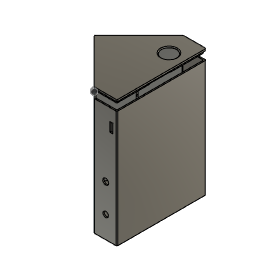
campanion enclosure (Autodesk Fusion 360 design; units mm, degrees)
Autodesk Fusion 360 part; units mm, degrees
note: some values were not read from the file. Chosen so that the rebuilt part matches the saved one: which face or edge a step refers to. Set by a fixed rule: which sketch regions a step uses.
sketch "Sketch1" plane through (0, 0, 0) normal (1, 0, 0) x (0, 1, 0)
  line L0 (0, 0) -> (51.6188, -51.6188)
  line L1 (0, 0) -> (73, 0) construction
  line L2 (0, 0) -> (0, -106.5194)
  line L3 (51.6188, -51.6188) -> (51.6188, -76.6188)
  line L4 (51.6188, -76.6188) -> (0, -76.6188)
  line L5 (0, 0) -> (-51.6188, -51.6188)
  line L6 (-51.6188, -51.6188) -> (-51.6188, -76.6188)
  line L7 (-51.6188, -76.6188) -> (0, -76.6188)
  line L8 (0, 2.1213) -> (53.1188, -50.9975)
  line L9 (53.1188, -50.9975) -> (53.1188, -78.1188)
  line L10 (53.1188, -78.1188) -> (0, -78.1188)
  line L11 (0, 2.1213) -> (-53.1188, -50.9975)
  line L12 (-53.1188, -50.9975) -> (-53.1188, -78.1188)
  line L13 (-53.1188, -78.1188) -> (0, -78.1188)
  dimension "d6" = 45
  dimension "d7" = 73
  dimension "d8" = 25
  constraint horizontal L1
  constraint coincident L0.start L1.start
  constraint perpendicular L1 L2
  constraint vertical L3
  constraint coincident L2 L4.end
  constraint perpendicular L2 L4
  constraint symmetric L0.start L2 L1.start
  constraint symmetric L0.end L2 L5.end
  constraint symmetric L2 L3.end L6.end
  constraint symmetric L2 L4.end L7.end
  constraint parallel L0 L8
  constraint parallel L3 L9
  constraint parallel L4 L10
  constraint parallel L5 L11
  constraint parallel L6 L12
  constraint parallel L7 L13
  measures "d6" angle of L0 L1
  measures "d7" distance of L0.start L0.end
  measures "d8" distance of L0.end L3.end
extrude "Extrude1" add sketch "Sketch1" along normal blind 124 makes body 1
sketch "Sketch3" plane through (0, -53.6188, 0) normal (0, -1, 0) x (1, 0, 0)
  line L0 (0, -78.6188) -> (124, -78.6188)
  line L1 (124, -78.6188) -> (124, -50.7904)
  line L2 (124, -50.7904) -> (0, -50.7904)
  line L3 (122.913, -78.6188) -> (122.913, -64.7048)
  line L4 (122.913, -64.7048) -> (124, -64.7046)
  line L5 (122.913, -64.7048) -> (-1, -64.7047)
  circle A0 centre (21.121, -64.7047) radius 3.25
  circle A1 centre (54.96, -64.7181) radius 3.5
  line L6 (124, -64.7046) -> (104.5, -64.7046)
  line L7 (-1, -64.7047) -> (18.5, -64.7047)
  line L8 (0, -50.7904) -> (0, -78.6188)
  dimension "d17" = 27.8284
  dimension "d18" = 13.914
  dimension "d19" = 6.5
  dimension "d20" = 7
  dimension "d21" = 19.5
  dimension "d22" = 19.5
  constraint coincident L0 L3.start
  constraint perpendicular L0 L3
  constraint midpoint L1 L4.end
  constraint coincident L5 A0.centre
  constraint coincident L4 A1.centre
  constraint perpendicular L1 L6
  measures "d17" distance of L0 L2
  measures "d18" distance of L3.start L3.end
  measures "d19" diameter of A0
  measures "d20" diameter of A1
  measures "d21" distance of L4.end L6.end
  measures "d22" distance of L5.end L7.end
extrude "Extrude3" cut sketch "Sketch3" against normal blind 2 contours L5 A0 L7 | L5 A0 L7 | L5 A1 | L5 A1 bodies 1
sketch "Sketch4" plane through (0, -1.4142, 1.4142) normal (0, -0.707107, 0.707107) x (1, 0, 0)
  line L0 (0, -73.8284) -> (124, -73.8284)
  line L1 (124, -73.8284) -> (124, 2)
  line L2 (124, 2) -> (0, 2)
  line L3 (1.4348, -7.7738) -> (77.4348, -7.7738)
  line L4 (77.4348, -7.7738) -> (77.4348, -62.7738)
  line L5 (77.4348, -62.7738) -> (1.4348, -62.7738)
  line L6 (1.4348, -62.7738) -> (1.4348, -7.7738)
  line L7 (0, 2) -> (0, -73.8284)
  dimension "d25" = 76
  dimension "d26" = 55
  constraint horizontal L3
  constraint vertical L4
  constraint horizontal L5
  constraint vertical L6
  measures "d25" distance of L3.start L3.end
  measures "d26" distance of L3.start L5.end
extrude "Extrude4" cut sketch "Sketch4" against normal blind 2 contours L3 L4 L5 L6 bodies 1
extrude "Extrude5" add 1 faces at (0, -17.2063, -77.6188) along direction (-1, 0, 0) blind 3 on bodies 1 bodies 1
ref_plane "WorkPlane1" through (-3, 0, 0) normal (1, 0, 0) x (0, 1, 0)
sketch "Sketch6" plane through (-3, 0, 0) normal (1, 0, 0) x (0, 1, 0)
  line L0 (0, 1.066) -> (-52.4214, -50.8821)
  line L1 (-52.4214, -50.8821) -> (-52.4214, -77.9172)
  line L2 (-52.4214, -77.9172) -> (52.8588, -77.9172)
  line L3 (52.8588, -77.9172) -> (52.8588, -50.8821)
  line L4 (52.8588, -50.8821) -> (0, 1.066)
  constraint vertical L1
  constraint perpendicular L1 L2
  constraint perpendicular L2 L3
extrude "Extrude7" add 1 faces at (-3, -17.2063, -77.6188) along direction (-1, 0, 0) blind 2 on bodies 1 bodies 1
extrude "Extrude8" add sketch "Sketch6" against normal blind 2 bodies 1
ref_plane "WorkPlane2" through (59.5, -1.4571, -49.5404) normal (0, -0.707107, 0.707107) x (0, -0.707107, -0.707107)
sketch "Sketch7" plane through (49.5, -1.3536, -49.4368) normal (0, -0.707107, 0.707107) x (0, -0.707107, -0.707107)
  line L0 (-37.4062, -54.4523) -> (37.8896, -54.4523)
  line L1 (37.8896, -54.4523) -> (37.8896, 74.4408)
  line L2 (37.8896, 74.4408) -> (-37.4062, 74.4408)
  line L3 (-37.4062, 74.4408) -> (-37.4062, -54.4523)
  constraint horizontal L0
  constraint vertical L1
  constraint horizontal L2
  constraint vertical L3
extrude "Extrude12" add 1 faces at (124, -17.2063, -77.6188) along direction (1, 0, 0) blind 10 on bodies 1 bodies 1
ref_plane "WorkPlane3" through (134, 0, 0) normal (1, 0, 0) x (0, 1, 0)
sketch "Sketch8" plane through (134, 0, 0) normal (1, 0, 0) x (0, 1, 0)
  line L0 (-27.0492, -74.4051) -> (-30.0877, -77.4712)
  line L1 (-30.0877, -77.4712) -> (-28.0645, -78.0602)
  line L2 (-25.4859, -75.6609) -> (-27.3218, -77.4968)
  line L3 (-27.3218, -77.4968) -> (-28.0645, -78.0602)
  line L4 (-27.0492, -74.4051) -> (-25.4859, -75.6609)
sketch "Sketch9" plane through (49.5, -1.3536, -49.4368) normal (0, -0.707107, 0.707107) x (0, -0.707107, -0.707107)
sketch "Sketch10" plane through (49.5, -1.3536, -49.4368) normal (0, -0.707107, 0.707107) x (0, -0.707107, -0.707107)
  line L0 (37.1723, -20.8219) -> (40.3659, -20.8219)
  line L1 (40.3659, -20.8219) -> (40.3659, -0.7333)
  line L2 (40.3659, -0.7333) -> (37.1723, -0.7333)
  line L3 (37.1723, -0.7333) -> (37.1723, -20.8219)
  line L4 (37.1723, 35.5294) -> (40.3659, 35.5294)
  line L5 (40.3659, 35.5294) -> (40.3659, 52.3215)
  line L6 (40.3659, 52.3215) -> (37.1723, 52.3215)
  line L7 (37.1723, 52.3215) -> (37.1723, 35.5294)
  constraint horizontal L0
  constraint vertical L1
  constraint horizontal L2
  constraint vertical L3
  constraint horizontal L4
  constraint vertical L5
  constraint horizontal L6
  constraint vertical L7
extrude "Extrude11" add sketch "Sketch10" along normal blind 18 bodies 1
fillet "Fillet1" radius 1 16 edges at (38.7224, -40.3663, -62.9937) (48.7667, -34.0023, -69.3576) (48.7667, -36.941, -70.9353) (48.7667, -41.4954, -64.1228) (38.7224, -42.6245, -65.2519) (28.6781, -41.4954, -64.1228) (28.6781, -36.941, -70.9353) (28.6781, -34.0023, -69.3576) (85.0294, -34.0023, -69.3576) (85.0294, -36.941, -70.9353) (85.0294, -41.4954, -64.1228) (93.4254, -42.6245, -65.2519) (93.4254, -40.3663, -62.9937) (101.8215, -34.0023, -69.3576) (101.8215, -36.941, -70.9353) (101.8215, -41.4954, -64.1228) on bodies 1
extrude "Extrude15" add sketch "Sketch7" against normal blind 1.5 bodies 1
extrude "Extrude16" add 1 faces at (123.9408, -10.1727, -58.9631) along direction (1, 0, 0) blind 6 on bodies 1 bodies 1
sketch "Sketch12" plane through (59.5, -1.4571, -49.5404) normal (0, -0.707107, 0.707107) x (0, -0.707107, -0.707107)
  arc A0 (26.953, 71.0768) -> (34.3847, 71.0214) centre (30.6697, 71.1648) ccw
  line L0 (26.953, 71.0768) -> (34.3847, 71.0214)
extrude "Extrude17" cut sketch "Sketch12" against normal blind 2 bodies 1
fillet "Fillet2" radius 1 2 edges at (129.9408, -25.1921, -74.336) (129.9408, -20.035, -69.1789) on bodies 1
ref_plane "WorkPlane4" through (130, 0, -37.9987) normal (1, 0, 0) x (0, 0, -1)
sketch "Sketch14" plane through (130, 0, -37.9987) normal (1, 0, 0) x (0, 1, 0)
  line L0 (-26.6567, -36.7204) -> (-25.4859, -37.6609)
  line L1 (-27.3218, -39.4968) -> (-28.0645, -40.0602)
  line L2 (-26.6567, -36.7204) -> (-29.5406, -39.6304)
  line L3 (-25.4859, -37.6609) -> (-27.3218, -39.4968)
  line L4 (-29.5406, -39.6304) -> (-28.0645, -40.0602)
extrude "Extrude18" add sketch "Sketch14" against normal blind 134 bodies 1
fillet "Fillet3" radius 1 3 edges at (65.5, -51.6188, -51.6188) (65.5, -51.6188, -76.6188) (65.5, 51.6188, -76.6188) on bodies 1
fillet "Fillet4" radius 1 5 edges at (64.5, -53.1188, -50.9975) (64.5, -53.1188, -78.1188) (64.5, 0, 2.1213) (64.5, 53.1188, -50.9975) (64.5, 53.1188, -78.1188) on bodies 1
move_body "Move2" bodies 1 to x (0, 0, 1) y (0, 1, 0) z (-1, 0, 0) at (56.8518, 20, -87.1482)
sketch "Sketch15" plane through (38.4259, 38.4259, 0) normal (0.707107, 0.707107, 0) x (-0.707107, 0.707107, 0)
  line L0 (-88.8319, -9.7134) -> (-33.8319, -9.7134)
  line L1 (-33.8319, -9.7134) -> (-33.8319, -85.7134)
  line L2 (-33.8319, -85.7134) -> (-88.8319, -85.7134)
  line L3 (-88.8319, -85.7134) -> (-88.8319, -9.7134)
  line L4 (-98.6439, 46.8518) -> (-98.6439, -90.1482)
  line L5 (-98.6439, -90.1482) -> (-26.0582, -90.1482)
  line L6 (-26.0582, -90.1482) -> (-26.0582, 46.8518)
  line L7 (-26.0582, 46.8518) -> (-98.6439, 46.8518)
  line L8 (-74.851, 46.8518) -> (-49.851, 46.8518)
  line L9 (-49.851, 46.8518) -> (-49.851, 43.8518)
  line L10 (-49.851, 43.8518) -> (-74.851, 43.8518)
  line L11 (-74.851, 43.8518) -> (-74.851, 46.8518)
  line L12 (-62.351, 46.8518) -> (-62.351, 43.8518)
  dimension "d71" = 3
  dimension "d77" = 25
  constraint horizontal L8
  constraint vertical L9
  constraint horizontal L10
  constraint vertical L11
  constraint coincident L7 L8.start
  constraint midpoint L7 L12.start
  constraint midpoint L10 L12.end
  constraint vertical L12
  measures "d71" distance of L8.start L10.end
  measures "d77" distance of L9.end L10.end
extrude "Extrude19" add sketch "Sketch15" along normal blind 8 draft -45 contours L7 L8 L10 L11 L12 | L7 L8 L9 L10 L12 bodies 1
ref_plane "WorkPlane5" through (120.6777, 20, -21.6482) normal (0, 1, 0) x (-1, 0, 0)
mirror "Mirror1" about plane through (120.6777, 20, -21.6482) normal (0, 1, 0) of "Extrude19"
sketch "Sketch16" plane through (133.4706, 0, 0) normal (-1, 0, 0) x (0, -1, 0)
  line L0 (-70.6188, 46.8518) -> (-70.6188, -90.1482)
  line L1 (-70.6188, -90.1482) -> (6.4142, -90.1482)
  line L2 (6.4142, -90.1482) -> (6.4142, 42.7926)
  line L3 (6.4142, 42.7926) -> (6.4451, 42.7926)
  line L4 (6.4451, 42.7926) -> (6.4451, 42.8518)
  line L5 (6.4451, 42.8518) -> (8.5393, 42.8518)
  line L6 (8.5393, 42.8518) -> (8.5393, 14.6733)
  line L7 (8.5393, 14.6733) -> (9.8433, 14.6733)
  ellipse E0 centre (9.8433, 13.6733) end of major axis (11.2576, 13.6733) minor radius 1 (11.2576, 13.6733) -> (9.8433, 14.6733) ccw
  line L8 (11.2576, 13.6733) -> (11.2576, -1.1188)
  ellipse E1 centre (9.8433, -1.1188) end of major axis (11.2576, -1.1188) minor radius 1 (9.8433, -2.1188) -> (11.2576, -1.1188) ccw
  line L9 (9.8433, -2.1188) -> (8.5393, -2.1188)
  line L10 (8.5393, -2.1188) -> (8.5393, -38.3815)
  line L11 (8.5393, -38.3815) -> (9.8433, -38.3815)
  ellipse E2 centre (9.8433, -39.3815) end of major axis (11.2576, -39.3815) minor radius 1 (11.2576, -39.3815) -> (9.8433, -38.3815) ccw
  line L12 (11.2576, -39.3815) -> (11.2576, -57.4701)
  ellipse E3 centre (9.8433, -57.4701) end of major axis (11.2576, -57.4701) minor radius 1 (9.8433, -58.4701) -> (11.2576, -57.4701) ccw
  line L13 (9.8433, -58.4701) -> (8.5393, -58.4701)
  line L14 (8.5393, -58.4701) -> (8.5393, -90.1482)
  line L15 (8.5393, -90.1482) -> (30.6188, -90.1482)
  line L16 (30.6188, -90.1482) -> (30.6188, 46.8518)
  line L17 (30.6188, 46.8518) -> (-70.6188, 46.8518)
  line L18 (-32.5, 46.8518) -> (-7.5, 46.8518)
  line L19 (-7.5, 46.8518) -> (-7.5, 43.8518)
  line L20 (-7.5, 43.8518) -> (-32.5, 43.8518)
  line L21 (-32.5, 43.8518) -> (-32.5, 46.8518)
  line L22 (-20, 46.8518) -> (-20, 43.8518) construction
  dimension "d82" = 3
  dimension "d83" = 25
  constraint horizontal L18
  constraint vertical L19
  constraint horizontal L20
  constraint vertical L21
  constraint coincident L17 L18.start
  constraint midpoint L17 L22.start
  constraint midpoint L20 L22.end
  constraint vertical L22
  measures "d82" distance of L18.start L20.end
  measures "d83" distance of L19.end L20.end
extrude "Extrude20" add sketch "Sketch16" along normal blind 8 draft -45 contours L17 L18 L19 L20 L21 bodies 1
fillet "Fillet5" radius 1 1 edges at (108.4706, 71.6188, -21.6482) on bodies 1
sketch "Sketch1 (2)" plane through (0, 0, 46.8518) normal (0, 0, 1) x (-1, 0, 0) in component "Top"
  arc A0 (-134.9706, -72.1188) -> (-133.9706, -73.1188) centre (-133.9706, -72.1188) ccw
  line L0 (-133.9706, -73.1188) -> (-108.2635, -73.1188)
  arc A1 (-108.2635, -73.1188) -> (-107.5564, -72.8259) centre (-108.2635, -72.1188) ccw
  line L1 (-107.5564, -72.8259) -> (-55.4376, -20.7071)
  arc A2 (-55.4376, -20.7071) -> (-55.4376, -19.2929) centre (-56.1447, -20) ccw
  line L2 (-55.4376, -19.2929) -> (-107.5564, 32.8259)
  arc A3 (-107.5564, 32.8259) -> (-108.2635, 33.1188) centre (-108.2635, 32.1188) ccw
  line L3 (-108.2635, 33.1188) -> (-133.9706, 33.1188)
  arc A4 (-133.9706, 33.1188) -> (-134.9706, 32.1188) centre (-133.9706, 32.1188) ccw
  line L4 (-134.9706, 32.1188) -> (-134.9706, -72.1188)
  line L5 (-108.1777, 31.3259) -> (-91.3536, 14.5018)
  line L6 (-91.3536, 14.5018) -> (-73.6759, -3.1759)
  line L7 (-73.6759, -3.1759) -> (-56.8518, -20)
  line L8 (-56.8518, -20) -> (-73.6759, -36.8241)
  line L9 (-73.6759, -36.8241) -> (-91.3536, -54.5018)
  line L10 (-91.3536, -54.5018) -> (-108.1777, -71.3259)
  arc A5 (-108.8848, -71.6188) -> (-108.1777, -71.3259) centre (-108.8848, -70.6188) ccw
  line L11 (-108.8848, -71.6188) -> (-132.4706, -71.6188)
  arc A6 (-133.4706, -70.6188) -> (-132.4706, -71.6188) centre (-132.4706, -70.6188) ccw
  line L12 (-133.4706, -70.6188) -> (-133.4706, -32.5)
  line L13 (-133.4706, -32.5) -> (-133.4706, -7.5)
  line L14 (-133.4706, -7.5) -> (-133.4706, 30.6188)
  arc A7 (-132.4706, 31.6188) -> (-133.4706, 30.6188) centre (-132.4706, 30.6188) ccw
  line L15 (-132.4706, 31.6188) -> (-108.8848, 31.6188)
  arc A8 (-108.1777, 31.3259) -> (-108.8848, 31.6188) centre (-108.8848, 30.6188) ccw
extrude "Extrude1'" add sketch "Sketch1 (2)" along normal blind 2 separate body contours A0 L0 A1 L1 A2 L2 A3 L3 A4 L4 | L5 L6 L7 L8 L9 L10 A5 L11 A6 L12 L13 L14 A7 L15 A8 makes body 2 in component "Top"
sketch "Sketch2" plane through (0, 0, 46.8518) normal (0, 0, -1) x (1, 0, 0) in component "Top"
  line L0 (134.9706, -72.1188) -> (134.9706, 32.1188)
  arc A0 (134.9706, 32.1188) -> (133.9706, 33.1188) centre (133.9706, 32.1188) ccw
  line L1 (133.9706, 33.1188) -> (108.2635, 33.1188)
  arc A1 (108.2635, 33.1188) -> (107.5564, 32.8259) centre (108.2635, 32.1188) ccw
  line L2 (107.5564, 32.8259) -> (55.4376, -19.2929)
  arc A2 (55.4376, -19.2929) -> (55.4376, -20.7071) centre (56.1447, -20) ccw
  line L3 (55.4376, -20.7071) -> (107.5564, -72.8259)
  arc A3 (107.5564, -72.8259) -> (108.2635, -73.1188) centre (108.2635, -72.1188) ccw
  line L4 (108.2635, -73.1188) -> (133.9706, -73.1188)
  arc A4 (133.9706, -73.1188) -> (134.9706, -72.1188) centre (133.9706, -72.1188) ccw
  line L5 (133.2706, 31.4188) -> (108.5534, 31.4188)
  line L6 (108.5534, 31.4188) -> (57.1346, -20)
  line L7 (57.1346, -20) -> (108.5534, -71.4188)
  line L8 (108.5534, -71.4188) -> (133.2706, -71.4188)
  line L9 (133.2706, -71.4188) -> (133.2706, 31.4188)
extrude "Extrude2" add sketch "Sketch2" along normal blind 3 contours L5 L6 L7 L8 L9 bodies 2 in component "Top"
extrude "Extrude3'" cut sketch "Sketch16" along normal blind 3 draft -45 from surface at 0.2 contours L17 L18 L19 L20 L21 bodies 2 in component "Top"
extrude "Extrude4'" cut sketch "Sketch15" along normal blind 3 draft -45 from surface at 0.2 contours L7 L8 L10 L11 L12 | L7 L8 L9 L10 L12 bodies 2 in component "Top"
mirror "Mirror1'" about plane through (120.6777, 20, -21.6482) normal (0, 1, 0) of "Extrude4'" in component "Top"
shell "Shell1" thickness 1.5 removed faces 1 at (93.6351, 15.8333, 43.8518) on bodies 2 in component "Top"
chamfer "Chamfer1" distance 0.6 angle 45 3 edges at (133.2706, 20, 43.8518) (82.6562, -5.5215, 43.8518) (82.6562, 45.5215, 43.8518) on bodies 2 in component "Top"
move_body "Move1" bodies 2 to x (1, 0, 0) y (0, 1, 0) z (0, 0, 1) at (0, 0, 10) in component "Top"
sketch "Sketch17" plane through (0, -33.1188, 0) normal (0, -1, 0) x (1, 0, 0)
  circle A0 centre (121.5565, -66.0272) radius 3.25
  circle A1 centre (121.5699, -32.1882) radius 3.5
  line L0 (133.9706, -92.1482) -> (133.9706, 46.8518)
  line L1 (133.9706, 46.8518) -> (108.2635, 46.8518)
  line L2 (108.2635, 46.8518) -> (108.2635, -92.1482)
  line L3 (108.2635, -92.1482) -> (133.9706, -92.1482)
  line L4 (126.5371, 21.3223) -> (130.0371, 21.3223)
  line L5 (130.0371, 21.3223) -> (130.0371, 32.3223)
  line L6 (130.0371, 32.3223) -> (126.5371, 32.3223)
  line L7 (126.5371, 32.3223) -> (126.5371, 21.3223)
  dimension "d103" = 11
  dimension "d104" = 3.5
  constraint horizontal L4
  constraint vertical L5
  constraint horizontal L6
  constraint vertical L7
  measures "d103" distance of L4.start L6.end
  measures "d104" distance of L4.start L4.end
extrude "Extrude21" cut sketch "Sketch17" against normal blind 2 contours L4 L5 L6 L7 bodies 1
sketch "Sketch3 (2)" plane through (0, 0, 58.8518) normal (0, 0, 1) x (-1, 0, 0) in component "Top"
  line L0 (-134.9706, 32.1188) -> (-134.9706, -72.1188)
  arc A0 (-134.9706, -72.1188) -> (-133.9706, -73.1188) centre (-133.9706, -72.1188) ccw
  line L1 (-133.9706, -73.1188) -> (-108.2635, -73.1188)
  arc A1 (-108.2635, -73.1188) -> (-107.5564, -72.8259) centre (-108.2635, -72.1188) ccw
  line L2 (-107.5564, -72.8259) -> (-55.4376, -20.7071)
  arc A2 (-55.4376, -20.7071) -> (-55.4376, -19.2929) centre (-56.1447, -20) ccw
  line L3 (-55.4376, -19.2929) -> (-107.5564, 32.8259)
  arc A3 (-107.5564, 32.8259) -> (-108.2635, 33.1188) centre (-108.2635, 32.1188) ccw
  line L4 (-108.2635, 33.1188) -> (-133.9706, 33.1188)
  arc A4 (-133.9706, 33.1188) -> (-134.9706, 32.1188) centre (-133.9706, 32.1188) ccw
  line L5 (-134.9706, -72.1188) -> (-81.497, 6.7665)
  circle A5 centre (-117.5016, -46.3482) radius 9
  dimension "d107" = 18
  constraint coincident L0.end A0.start
  constraint midpoint L3 L5.end
  constraint coincident L5 A5.centre
  measures "d107" diameter of A5
extrude "Extrude5'" cut sketch "Sketch3 (2)" against normal blind 3 contours L5 A5 | L5 A5 bodies 2 in component "Top"
fillet "Fillet1'" radius 1 1 edges at (125.8926, 43.0937, 58.8518) on bodies 2 in component "Top"
fillet "Fillet2'" radius 1 1 edges at (125.8926, 49.6028, 57.3518) on bodies 2 in component "Top"
sketch "Sketch18" plane through (37.3652, 37.3652, 0) normal (-0.707107, -0.707107, 0) x (0.707107, -0.707107, 0)
  line L0 (25.5582, 46.8518) -> (25.5582, -92.1482)
  line L1 (25.5582, -92.1482) -> (99.2653, -92.1482)
  line L2 (99.2653, -92.1482) -> (99.2653, 46.8518)
  line L3 (99.2653, 46.8518) -> (25.5582, 46.8518)
  line L4 (33.8319, -9.7134) -> (88.8319, -9.7134)
  line L5 (88.8319, -9.7134) -> (88.8319, -85.7134)
  line L6 (88.8319, -85.7134) -> (33.8319, -85.7134)
  line L7 (33.8319, -85.7134) -> (33.8319, -9.7134)
  arc A0 (86.6151, 46.8518) -> (90.2437, 46.8518) centre (88.4294, 46.8518) ccw
  line L8 (86.6151, 46.8518) -> (90.2437, 46.8518)
  constraint coincident L3 A0.end
  constraint coincident L3 A0.centre
  constraint parallel L3 L8
extrude "Extrude22" cut sketch "Sketch18" against normal blind 2 contours L3 A0 L8 bodies 1
move_body "Move2'" [suppressed] in component "Top"
component "Top" placed x (1, 0, 0) y (0, 1, 0) z (0, 0, 1) at (0, 0, 0)
equation "d18 = ( 27.828 / 2 ) * 1 mm"
equation "d71 = shell * 2"
equation "width = 50 mm"
equation "length = 50 mm"
equation "height = 25 mm"
equation "shell = 1.5 mm"
equation "gap = 0.2 mm"
equation "d77 = width / 2"
equation "d82 = shell * 2"
equation "d83 = width / 2"
equation "d90 = -( shell + gap )"
equation "d91 = shell * 2"
equation "d94 = shell * 2"
equation "d97 = shell * 2"
equation "d101 = shell"
